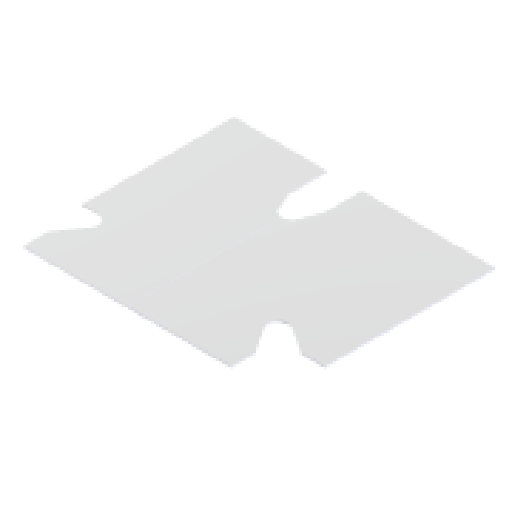
# Autodesk Inventor part: Electronics Cover Panel
Saved by Autodesk Inventor 2023.2 (Build 272271000, 271)
## iProperties
Created: 2023-02-24
Part Number: Electronics Cover Panel
Material: Aluminum 6061
Document SubType Name: Modeling
Designer: remop
Density: 2.7 g/cm^3
Appearance: Aluminum - Flat
Author: remop
Autodesk Inventor part; units mm, degrees
ref_plane "YZ Plane" through (0, 0, 0) normal (1, 0, 0) x (0, 1, 0)
ref_plane "XZ Plane" through (0, 0, 0) normal (0, 1, 0) x (-1, 0, 0)
ref_plane "XY Plane" through (0, 0, 0) normal (0, 0, 1) x (1, 0, 0)
sketch "Sketch13" plane through (0, 0, 0) normal (0, 0, 1) x (1, 0, 0)
  line L0 (-25, -5) -> (-25, 5) projected
  line L1 (25, -5) -> (-25, -5) projected
  line L2 (25, 5) -> (25, -5) projected
  line L3 (-25, 5) -> (25, 5) projected
  line L4 (143.1641, 77.0898) -> (171.8171, 34.7554) projected
  arc A0 (167.4656, 101.3913) -> (143.1641, 77.0898) centre (157.6566, 86.8988) ccw projected
  line L5 (209.8, 72.7382) -> (167.4656, 101.3913) projected
  line L6 (227.0605, 72.7382) -> (209.8, 72.7382) projected
  arc A1 (227.0605, 72.7382) -> (224.4218, 74.9169) centre (214.3326, 60.0103) ccw projected
  line L7 (173.0707, 109.6728) -> (224.4218, 74.9169) projected
  arc A2 (173.0707, 109.6728) -> (134.8826, 71.4847) centre (157.6566, 86.8988) ccw projected
  line L8 (169.6384, 20.1336) -> (134.8826, 71.4847) projected
  arc A3 (169.6384, 20.1336) -> (171.8171, 17.4949) centre (184.5451, 30.2228) ccw projected
  line L9 (171.8171, 34.7554) -> (171.8171, 17.4949) projected
  line L10 (224.5554, 355) -> (224.5554, 345) projected
  line L11 (174.5554, 355) -> (224.5554, 355) projected
  line L12 (174.5554, 345) -> (174.5554, 355) projected
  line L13 (224.5554, 345) -> (174.5554, 345) projected
  line L14 (16.2119, 260.9456) -> (28.4741, 291.112) projected
  arc A4 (-16.2118, 260.9456) -> (16.2119, 260.9456) centre (0.0001, 267.5355) ccw projected
  line L15 (-28.474, 291.112) -> (-16.2118, 260.9456) projected
  arc A5 (-29.0629, 294.1245) -> (-28.474, 291.112) centre (-21.0629, 294.1245) ccw projected
  line L16 (-29.0629, 355) -> (-29.0629, 294.1245) projected
  line L17 (-41.0629, 355) -> (-29.0629, 355) projected
  line L18 (-41.0629, 294.1245) -> (-41.0629, 355) projected
  arc A6 (-41.0629, 294.1245) -> (-39.5907, 286.5932) centre (-21.0629, 294.1245) ccw projected
  line L19 (-27.3284, 256.4268) -> (-39.5907, 286.5932) projected
  arc A7 (-27.3284, 256.4268) -> (27.3286, 256.4268) centre (0.0001, 267.5355) ccw projected
  line L20 (39.5908, 286.5932) -> (27.3286, 256.4268) projected
  arc A8 (39.5908, 286.5932) -> (41.063, 294.1245) centre (21.063, 294.1245) ccw projected
  line L21 (41.063, 355) -> (41.063, 294.1245) projected
  line L22 (29.063, 355) -> (41.063, 355) projected
  line L23 (29.063, 294.1245) -> (29.063, 355) projected
  arc A9 (28.4741, 291.112) -> (29.063, 294.1245) centre (21.063, 294.1245) ccw projected
  line L24 (-128.4211, 355) -> (-128.4211, 345) projected
  line L25 (-178.4211, 355) -> (-128.4211, 355) projected
  line L26 (-178.4211, 345) -> (-178.4211, 355) projected
  line L27 (-128.4211, 345) -> (-178.4211, 345) projected
  line L28 (-183.4211, 104.3988) -> (-158.5223, 104.3988) projected
  arc A10 (-144.0298, 77.0898) -> (-158.5223, 104.3988) centre (-158.5223, 86.8988) ccw projected
  line L29 (-144.0298, 77.0898) -> (-172.6829, 34.7554) projected
  line L30 (-172.6829, 34.7554) -> (-172.6829, 17.4949) projected
  arc A11 (-172.6829, 17.4949) -> (-170.5041, 20.1336) centre (-185.4108, 30.2228) ccw projected
  line L31 (-170.5041, 20.1336) -> (-135.7483, 71.4847) projected
  arc A12 (-135.7483, 71.4847) -> (-158.5223, 114.3988) centre (-158.5223, 86.8988) ccw projected
  line L32 (-158.5223, 114.3988) -> (-183.4211, 114.3988) projected
  line L33 (-183.4211, 114.3988) -> (-183.4211, 104.3988) projected
  line L34 (-183.4211, 114.3988) -> (-183.4211, 355)
  line L35 (-183.4211, 355) -> (-178.4211, 355)
  line L36 (-128.4211, 355) -> (-41.0629, 355)
  line L37 (41.063, 355) -> (174.5554, 355)
  line L38 (224.5554, 355) -> (249.5554, 355)
  line L39 (249.5554, 355) -> (249.5554, 72.7382)
  line L40 (249.5554, 72.7382) -> (227.0605, 72.7382)
  line L41 (264.5554, -5) -> (264.5554, 355) projected
  line L42 (-25, -5) -> (-172.6829, -5)
  line L43 (-172.6829, -5) -> (-172.6829, 17.4949)
  line L44 (171.8171, 17.4949) -> (171.8171, -5)
  line L45 (171.8171, -5) -> (25, -5)
  line L46 (0.5001, 250.0427) -> (0.5001, -5)
  line L47 (-0.4999, 250.0427) -> (-0.4999, -5)
  line L48 (-265.4446, 355) -> (-265.4446, -5) projected
  line L49 (-250.4446, 325) -> (-250.4446, 355)
  line L50 (-250.4446, 355) -> (-183.4211, 355)
  line L51 (-250.4446, 325) -> (-183.4211, 325)
  circle A13 centre (142.8826, 68.4847) radius 1.45 projected
  circle A14 centre (176.0707, 101.6728) radius 1.45 projected
  circle A15 centre (-143.7483, 68.4847) radius 1.45 projected
  circle A16 centre (-163.5223, 109.3988) radius 1.45 projected
  circle A17 centre (-36.0629, 294.1245) radius 1.45 projected
  circle A18 centre (36.063, 294.1245) radius 1.45 projected
  circle A19 centre (-138.4211, 350) radius 1.45 projected
  circle A20 centre (-168.4211, 350) radius 1.45 projected
  circle A21 centre (214.5554, 350) radius 1.45 projected
  circle A22 centre (184.5554, 350) radius 1.45 projected
  circle A23 centre (-15, 0) radius 1.45 projected
  circle A24 centre (15, 0) radius 1.45 projected
  point P0 (0, 0)
  dimension "d27" = 15
  dimension "d28" = 1
  dimension "d31" = 15
  dimension "d32" = 30
  constraints: 32 end point, 7 perpendicular, 5 point on line, 3 collinear, 2 horizontal, 2 parallel, 2 point on circle, 2 vertical
  measures "d27" distance between parallel lines of L41 L39
  measures "d28" distance between parallel lines of L46 L47
  measures "d31" distance between parallel lines of L48 L49
  measures "d32" distance of L49.start L49.end
extrude "Extrusion14" add sketch "Sketch13" along normal blind 3 contours L42 L43 A11 L31 A12 L32 L34 L35 L26 L27 L24 L36 L18 A6 L19 A7 L47 L3 L0 | L0 L3 L47 L1 | L46 L3 L2 L1 | L30 L29 A10 L28 L33 L32 A12 L31 A11 | L46 A7 L20 A8 L21 L37 L12 L13 L10 L38 L39 L40 A1 L7 A2 L8 A3 L44 L45 L2 L3 | A7 L19 A6 L18 L17 L16 A5 L15 A4 L47 | L46 A4 L14 A9 L23 L22 L21 A8 L20 A7 | A3 L8 A2 L7 A1 L6 L5 A0 L4 L9 | L24 L27 L26 L25 | L11 L10 L13 L12
body "Solid11"
